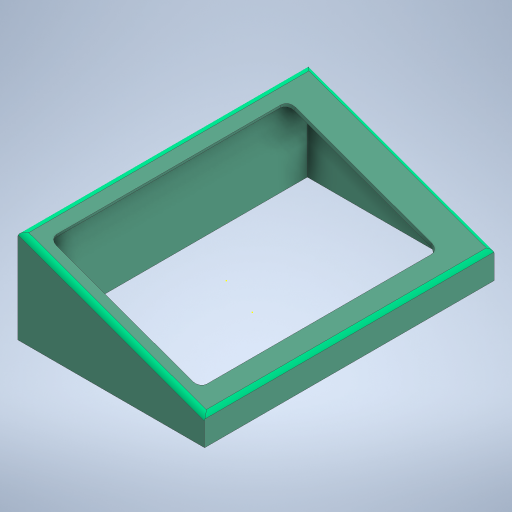
# Autodesk Inventor part: Screen_Support
Saved by Autodesk Inventor 2024 (Build 280153000, 153)
## iProperties
Created: 2024-02-15
Part Number: Screen_Support
Material: Generic
Document SubType Name: Modeling
Designer: fabiancastano
Density: 1 g/cm^3
Appearance: Default
Author: fabiancastano
Autodesk Inventor part; units mm, degrees
ref_plane "YZ Plane" through (0, 0, 0) normal (1, 0, 0) x (0, 1, 0)
sketch "Sketch1" plane through (0, 0, 0) normal (0, 1, 0) x (-1, 0, 0)
  line L0 (100, 155) -> (-100, 155)
  line L1 (-100, 155) -> (-100, -155)
  line L2 (-100, -155) -> (100, -155)
  line L3 (100, -155) -> (100, 155)
  point P0 (0, 0)
  point P1 (100, 0)
  point P2 (0, -155)
  dimension "d0" = 310
  dimension "d1" = 200
  constraints: 8 end point, 2 midpoint, 2 parallel, 1 horizontal, 1 horizontal alignment, 1 perpendicular, 1 vertical alignment
  measures "d0" distance of L2.end L0.start
  measures "d1" distance of L1.end L2.end
sketch "Sketch2" plane through (0, 0, 0) normal (0, 0, 1) x (1, 0, 0)
  line L0 (-100, 0) -> (100, 0)
  line L1 (100, 0) -> (100, 30)
  line L2 (100, 30) -> (-100, 102.794)
  line L3 (-100, 0) -> (-100, 102.794)
  line L4 (-96, 97.0815) -> (96, 27.1992)
  line L5 (96, 27.1992) -> (96, 0)
  line L6 (-96, 0) -> (-96, 97.0815)
  point P0 (0, 0)
  point P1 (0, 0)
  dimension "d2" = 200
  dimension "d3" = 30
  dimension "d4" = 110
  dimension "d5" = 4
  dimension "d6" = 110
  dimension "d7" = 4
  dimension "d8" = 27.1992
  constraints: 14 end point, 2 coincident, 2 point on line, 2 vertical, 1 horizontal, 1 midpoint
  measures "d2" distance of L0.start L0.end
  measures "d3" distance of L0.end L1.end
  measures "d4" angle of L2 L1
  measures "d5" distance between parallel lines of L3 L6
  measures "d6" angle of L5 L4
  measures "d7" distance between parallel lines of L1 L5
  measures "d8" distance of L4.end L5.end
extrude "Extrusion1" add sketch "Sketch2" along normal mid plane 310
extrude "Extrusion2" cut sketch "Sketch2" along normal mid plane 302 contours L6 L4 L5 L0
sketch "Sketch3" plane through (-100, 102.794, 155) normal (0.3420201, 0.9396926, 0) x (0.9396926, -0.3420201, 0)
  line L0 (27.85, 15) -> (183.2, 15)
  line L1 (191.05, 22.85) -> (191.05, 263.3)
  line L2 (183.2, 271.15) -> (27.85, 271.15)
  line L3 (20, 263.3) -> (20, 22.85)
  line L4 (0, 310) -> (0, 0) projected
  line L5 (212.8356, 0) -> (0, 0) projected
  arc A0 (20, 22.85) -> (27.85, 15) centre (27.85, 22.85) ccw
  arc A1 (27.85, 271.15) -> (20, 263.3) centre (27.85, 263.3) ccw
  arc A2 (191.05, 263.3) -> (183.2, 271.15) centre (183.2, 263.3) ccw
  arc A3 (183.2, 15) -> (191.05, 22.85) centre (183.2, 22.85) ccw
  point P0 (129.1269, 155)
  point P1 (191.05, 271.15)
  point P2 (191.05, 15)
  point P3 (20, 271.15)
  dimension "d13" = 171.05
  dimension "d14" = 256.15
  dimension "d15" = 20
  dimension "d16" = 15
  dimension "d17" = 7.85
  dimension "d18" = 7.85
  constraints: 8 end point, 8 point on circle, 8 tangent, 6 point on line, 4 centre point, 2 equal radius, 2 parallel, 1 horizontal, 1 perpendicular
  measures "d13" distance of point (20, 271.15) point (191.05, 271.15)
  measures "d14" distance of point (191.05, 271.15) point (191.05, 15)
  measures "d15" distance between parallel lines of L4 L3
  measures "d16" distance between parallel lines of L5 L0
  measures "d17" radius of A0
  measures "d18" radius of A1
extrude "Extrusion3" cut sketch "Sketch3" against normal up to next
fillet "Fillet1" radius 5 4 edges at (0, 66.397, 155) (0, 66.397, -155) (-100, 102.794, 0) (100, 30, 0)
ref_plane "Work Plane1" through (-10.2594, 70.1311, 132.15) normal (0.9396926, -0.3420201, 0) x (0, 0, -1)
sketch "Sketch4" plane through (-10.2594, 70.1311, 132.15) normal (0.9396926, -0.3420201, 0) x (0, 0, -1)
  point P0 (132.15, -62.3928)
ref_plane "Work Plane2" through (72.1517, 40.136, 4) normal (0, 0, -1) x (-0.9396926, 0.3420201, 0)
sketch "Sketch5" plane through (72.1517, 40.136, 4) normal (0, 0, -1) x (-0.9396926, 0.3420201, 0)
  point P0 (54.0731, -62.3928)
fillet "Fillet2" radius 3 1 edges at (-96, 97.0815, 0)
body "Solid1"
